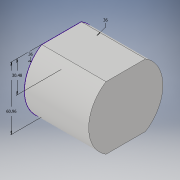
# Autodesk Inventor part: BattleBotmotormock
Saved by Autodesk Inventor 2019 (Build 230136000, 136)
## iProperties
Created: 2018-08-02
Part Number: BattleBotmotormock
Material: Generic
Document SubType Name: Modeling
Designer: Kitte_X
Density: 1 g/cm^3
Appearance: Default
Author: Kitte_X
Autodesk Inventor part; units mm, degrees
ref_plane "YZ Plane" through (0, 0, 0) normal (1, 0, 0) x (0, 1, 0)
ref_plane "XZ Plane" through (0, 0, 0) normal (0, 1, 0) x (-1, 0, 0)
ref_plane "XY Plane" through (0, 0, 0) normal (0, 0, 1) x (1, 0, 0)
sketch "Sketch1" plane through (0, 0, 0) normal (1, 0, 0) x (0, 1, 0)
  line L0 (30.48, 19.1565) -> (30.48, -19.1565)
  line L1 (-30.48, -19.1565) -> (-30.48, 19.1565)
  arc A0 (30.48, 19.1565) -> (-30.48, 19.1565) centre (0, 0) ccw
  arc A1 (-30.48, -19.1565) -> (30.48, -19.1565) centre (0, 0) ccw
  dimension "d1" = 60.96
  dimension "d2" = 30.48
  dimension "d3" = 36
  dimension "d4" = 36
  constraints: 4 end point, 4 point on circle, 2 centre point, 1 coincident, 1 parallel, 1 vertical
  measures "d1" distance between parallel lines of L1 L0
  measures "d2" distance from line of L0 point (0, 0)
  measures "d3" radius of A1
  measures "d4" radius of A0
extrude "Extrusion1" add sketch "Sketch1" along normal blind 62.5
body "Solid1"
